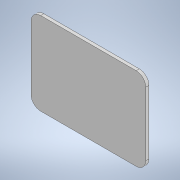
# Autodesk Inventor part: fleet_top
Saved by Autodesk Inventor 2020 (Build 240168000, 168)
## iProperties
Created: 2020-01-06
Part Number: fleet_top
Material: Generic
Document SubType Name: Modeling
Designer: my
Density: 1 g/cm^3
Appearance: Default
Author: my
Autodesk Inventor part; units mm, degrees
ref_plane "YZ Plane" through (0, 0, 0) normal (1, 0, 0) x (0, 1, 0)
ref_plane "XZ Plane" through (0, 0, 0) normal (0, 1, 0) x (-1, 0, 0)
ref_plane "XY Plane" through (0, 0, 0) normal (0, 0, 1) x (1, 0, 0)
sketch "Sketch1" plane through (0, 0, 0) normal (0, 0, 1) x (1, 0, 0)
  line L0 (-75, -65) -> (75, -65)
  line L1 (90, -50) -> (90, 50)
  line L2 (75, 65) -> (-75, 65)
  line L3 (-90, 50) -> (-90, -50)
  line L4 (-90, -65) -> (90, 65) construction
  line L5 (90, -65) -> (-90, 65) construction
  arc A0 (-75, 65) -> (-90, 50) centre (-75, 50) ccw
  arc A1 (-90, -50) -> (-75, -65) centre (-75, -50) ccw
  arc A2 (75, -65) -> (90, -50) centre (75, -50) ccw
  arc A3 (90, 50) -> (75, 65) centre (75, 50) ccw
  point P0 (0, 0)
  dimension "d0" = 130
  dimension "d1" = 180
  dimension "d2" = 15
  dimension "d3" = 15
  constraints: 12 end point, 8 point on circle, 8 point on line, 8 tangent, 4 centre point, 2 equal radius, 2 midpoint, 2 parallel, 1 horizontal, 1 perpendicular
  measures "d0" distance of L5.start L4.end
  measures "d1" distance of L4.end L5.end
  measures "d2" radius of A0
  measures "d3" radius of A1
extrude "Extrusion1" add sketch "Sketch1" along normal blind 5
body "Solid1"
